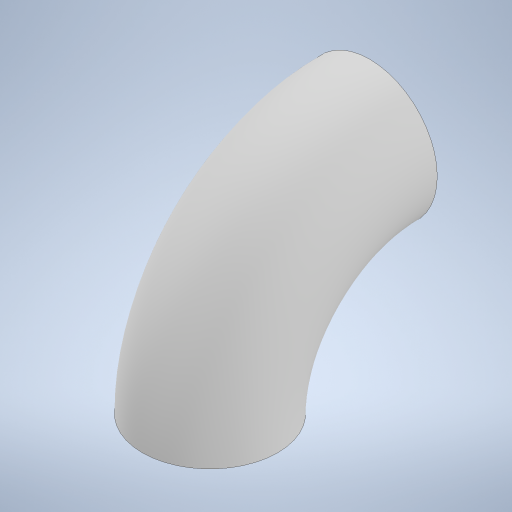
# Autodesk Inventor part: 06-01-2023 curva 90°
Saved by Autodesk Inventor 2023 (Build 270158000, 158)
## iProperties
Created: 2023-05-31
Part Number: 06-01-2023 curva 90°
Material: Generico
Document SubType Name: Modeling
Designer: Admin
Density: 1 g/cm^3
Appearance: Default
Author: Admin
Autodesk Inventor part; units mm, degrees
ref_plane "YZ Plane" through (0, 0, 0) normal (1, 0, 0) x (0, 1, 0)
ref_plane "XZ Plane" through (0, 0, 0) normal (0, 1, 0) x (-1, 0, 0)
ref_plane "XY Plane" through (0, 0, 0) normal (0, 0, 1) x (1, 0, 0)
sketch "Schizzo1" plane through (0, 0, 0) normal (0, 1, 0) x (-1, 0, 0)
  circle A0 centre (0, 0) radius 24.15
  circle A1 centre (0, 0) radius 22.65
  dimension "d0" = 48.3
  dimension "d1" = 45.3
  constraints: 2 centre point, 2 coincident
  measures "d0" diameter of A0
  measures "d1" diameter of A1
sketch "Schizzo2" plane through (0, 0, 0) normal (1, 0, 0) x (0, 1, 0)
  arc A0 (57, -57) -> (0, 0) centre (0, -57) ccw
  line L0 (0, -57) -> (57, -57) construction
  line L1 (0, -57) -> (0, 0) construction
  dimension "d2" = 90
  dimension "d4" = 57
  constraints: 4 end point, 2 point on circle, 1 centre point, 1 vertical alignment
  measures "d2" angle of L0 L1
  measures "d4" radius of A0
sweep "Sweep1" add profiles "Schizzo1" path "Schizzo2"
